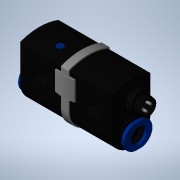
# Autodesk Inventor part: 527458 SDE5-Q6-M8(O)---(DS)
Saved by Autodesk Inventor 2021 (Build 250183000, 183)
## iProperties
Created: 2026-04-21
Part Number: 527458 SDE5-Q6-M8(O)---(DS)
Material: Generic
Catalog Web Link: www.3dfindit.com
Description: SDE5-(DS)-Pressure sensors - Housing
Vendor: FESTO
Document SubType Name: Modeling
Designer: psAdmin
Manufacturer: FESTO
Mass: 14.2277 g
Surface Area: 44.8821 cm^2
Volume: 14.2277 cm^3
Density: 1 g/cm^3
Appearance: PSOLRGB-79-79-79
Category: PARTsolutions
Company: FESTO
Title: 527458 SDE5-Q6-M8(O)---(DS)
Author: Cadenas PARTsolutions
Comments: Pressure sensors - Housing
PSOL_IDENT_0: {$CADENAS_DATA/23d-libs/festo/parts/s/sde5/parts/sde5.prj},216 {VTYP=3D},{NB=527458 SDE5-Q6-M8(O)---
PSOL_IDENT_1: (DS)},{LINA=527458 SDE5-Q6-M8(O)---(DS)},{NN=SDE5-(DS)},{DATE=22.08.2025 13:16:38},{GEOMDATE=30.08.2
PSOL_IDENT_2: 023 07:21:38},{VERSION=},{LINEID=110},{WBVAR=SF,PA,EAN,WSEX},{WBNUMERIC=WSEX}  {NB=527458 SDE5-Q6-M8
PSOL_IDENT_3: (O)---(DS)},{LINA=527458 SDE5-Q6-M8(O)---(DS)},{KT=DUMMY},{TNR=527458},{TYP=SDE5},{SF=O},{PA=Q6},{EA
PSOL_IDENT_4: N=M8},{PA1='Q6'},{PAN=1},{EA=P},{EAN1='M8'},{AK1=''},{VERS=11.000},{QST=3.1},{QSD=6},{EANX=2},{WSEX=
PSOL_IDENT_5: 0.000},{WSEX1=0.000},{WSEX2=}
NB: 527458 SDE5-Q6-M8(O)---(DS)
NN: SDE5-(DS)
NT: Pressure sensors - Housing
NBSYN: $TNR. $TYP.-$PA.-$EAN.($SF.)$WSEX2.---(DS)
LINA: 527458 SDE5-Q6-M8(O)---(DS)
CATALOG: Festo
TNR: 527458
TYP: SDE5
SF: O
PA: Q6
EAN: M8
EA: P
WSEX: 0
SUPPLIER: FESTO
ARTICLENO: 527458 SDE5-Q6-M8(O)---(DS)
BOMINFO: 527458 SDE5-Q6-M8(O)---(DS)
CREATOR: CADENAS GmbH
Autodesk Inventor part; units mm, degrees
sketch "Skizze_1" plane through (0, 0, 0) normal (1, 0, 0) x (0, 1, 0)
  arc A0 (8, 8) -> (8, -8) centre (8, 0) ccw
  line L0 (8, -8) -> (22.6494, -8)
  arc A1 (22.6494, -8) -> (23.118, -7.6744) centre (22.6494, -7.5) ccw
  arc A2 (23.118, -7.6744) -> (23.118, 7.6744) centre (2.5, 0) ccw
  arc A3 (23.118, 7.6744) -> (22.6494, 8) centre (22.6494, 7.5) ccw
  line L1 (22.6494, 8) -> (8, 8)
  constraints: 8 point on circle, 4 centre point, 4 end point
extrude "Extrusion1" add sketch "Skizze_1" along normal mid plane 38.5
sketch "Skizze_2" plane through (0, 0, 0) normal (0, 1, 0) x (-1, 0, 0)
  line L0 (0, -18) -> (0, -8)
  line L1 (0, -8) -> (-18.75, -8)
  arc A0 (-19.25, -7.5) -> (-18.75, -8) centre (-18.75, -7.5) ccw
  line L2 (-19.25, -7.5) -> (-19.25, 7.5)
  arc A1 (-18.75, 8) -> (-19.25, 7.5) centre (-18.75, 7.5) ccw
  line L3 (-18.75, 8) -> (0, 8)
  line L4 (0, 8) -> (0, 18)
  line L5 (0, 18) -> (-29.25, 18)
  line L6 (-29.25, 18) -> (-29.25, -18)
  line L7 (-29.25, -18) -> (0, -18)
  constraints: 16 end point, 4 point on circle, 2 centre point
extrude "Extrusion2" cut sketch "Skizze_2" along normal blind 25
sketch "Skizze_3" plane through (0, 0, 0) normal (0, 1, 0) x (-1, 0, 0)
  line L0 (29.25, -18) -> (29.25, 18)
  line L1 (29.25, 18) -> (0, 18)
  line L2 (0, 18) -> (0, 8)
  line L3 (0, 8) -> (18.75, 8)
  arc A0 (19.25, 7.5) -> (18.75, 8) centre (18.75, 7.5) ccw
  line L4 (19.25, 7.5) -> (19.25, -7.5)
  arc A1 (18.75, -8) -> (19.25, -7.5) centre (18.75, -7.5) ccw
  line L5 (18.75, -8) -> (0, -8)
  line L6 (0, -8) -> (0, -18)
  line L7 (0, -18) -> (29.25, -18)
  constraints: 16 end point, 4 point on circle, 2 centre point
extrude "Extrusion3" cut sketch "Skizze_3" along normal blind 25
sketch "Skizze_4" plane through (0, 0, 0) normal (0, 0, 1) x (1, 0, 0)
  line L0 (-2, 8) -> (2, 8)
  line L1 (-25, 3) -> (-25, -5.0034)
  line L2 (-25, -5.0034) -> (-14, -5.0034)
  line L3 (-14, -5.0034) -> (-14, 0)
  line L4 (-14, 0) -> (-18.75, 0)
  arc A0 (-19.25, 0.5) -> (-18.75, 0) centre (-18.75, 0.5) ccw
  line L5 (-19.25, 0.5) -> (-19.25, 3)
  line L6 (-19.25, 3) -> (-25, 3)
  constraints: 14 end point, 2 point on circle, 1 centre point
revolve "Revolution1" cut sketch "Skizze_4" angle 180 mid plane about axis through (-2, 8, 0) along (1, 0, 0)
sketch "Skizze_5" plane through (0, 0, 0) normal (0, 0, 1) x (1, 0, 0)
  line L0 (-2, 8) -> (2, 8)
  line L1 (14, -5.0034) -> (25, -5.0034)
  line L2 (25, -5.0034) -> (25, 3)
  line L3 (25, 3) -> (19.25, 3)
  line L4 (19.25, 3) -> (19.25, 0.5)
  arc A0 (18.75, 0) -> (19.25, 0.5) centre (18.75, 0.5) ccw
  line L5 (18.75, 0) -> (14, 0)
  line L6 (14, 0) -> (14, -5.0034)
  constraints: 14 end point, 2 point on circle, 1 centre point
revolve "Revolution2" cut sketch "Skizze_5" angle 180 mid plane about axis through (-2, 8, 0) along (1, 0, 0)
sketch "Skizze_6" plane through (0, 0, 0) normal (0, 0, 1) x (1, 0, 0)
  line L0 (-19.25, 2.5) -> (-24.25, 2.5)
  line L1 (-24.25, 29.5) -> (-24.25, 22.5)
  line L2 (-24.25, 22.5) -> (-19.25, 22.5)
  line L3 (-19.25, 22.5) -> (-19.25, 24)
  arc A0 (-18.75, 24.5) -> (-19.25, 24) centre (-18.75, 24) ccw
  line L4 (-18.75, 24.5) -> (-18.75, 29.5)
  line L5 (-18.75, 29.5) -> (-24.25, 29.5)
  constraints: 12 end point, 2 point on circle, 1 centre point
revolve "Revolution3" cut sketch "Skizze_6" angle 90 mid plane about axis through (-19.25, 2.5, 0) along (-1, 0, 0)
sketch "Skizze_7" plane through (0, 0, 0) normal (0, 0, 1) x (1, 0, 0)
  line L0 (24.25, 2.5) -> (19.25, 2.5)
  arc A0 (19.25, 24) -> (18.75, 24.5) centre (18.75, 24) ccw
  line L1 (19.25, 24) -> (19.25, 22.5)
  line L2 (19.25, 22.5) -> (24.25, 22.5)
  line L3 (24.25, 22.5) -> (24.25, 29.5)
  line L4 (24.25, 29.5) -> (18.75, 29.5)
  line L5 (18.75, 29.5) -> (18.75, 24.5)
  constraints: 12 end point, 2 point on circle, 1 centre point
revolve "Revolution4" cut sketch "Skizze_7" angle 90 mid plane about axis through (24.25, 2.5, 0) along (-1, 0, 0)
sketch "Skizze_8" plane through (-13.7, 0, 0) normal (1, 0, 0) x (0, 0, -1)
  line L0 (-10, 17) -> (-10, 10)
  line L1 (-10, 10) -> (-8, 10)
  line L2 (-8, 10) -> (-8, 12.0163)
  arc A0 (-7.6294, 12.4993) -> (-8, 12.0163) centre (-7.5, 12.0163) ccw
  line L3 (-7.6294, 12.4993) -> (-6.4224, 12.8227)
  arc A1 (-6.4224, 12.8227) -> (-6.2, 13.1125) centre (-6.5, 13.1125) ccw
  line L4 (-6.2, 13.1125) -> (-6.2, 14.8875)
  arc A2 (-6.2, 14.8875) -> (-6.4224, 15.1773) centre (-6.5, 14.8875) ccw
  line L5 (-6.4224, 15.1773) -> (-7.6294, 15.5007)
  arc A3 (-8, 15.9837) -> (-7.6294, 15.5007) centre (-7.5, 15.9837) ccw
  line L6 (-8, 15.9837) -> (-8, 17)
  line L7 (-8, 17) -> (-10, 17)
  constraints: 16 end point, 8 point on circle, 4 centre point
extrude "Extrusion4" cut sketch "Skizze_8" along normal blind 5.3
sketch "Skizze_9" plane through (-13.7, 0, 0) normal (1, 0, 0) x (0, 0, -1)
  line L0 (6.2, 14.8875) -> (6.2, 13.1125)
  arc A0 (6.2, 13.1125) -> (6.4224, 12.8227) centre (6.5, 13.1125) ccw
  line L1 (6.4224, 12.8227) -> (7.6294, 12.4993)
  arc A1 (8, 12.0163) -> (7.6294, 12.4993) centre (7.5, 12.0163) ccw
  line L2 (8, 12.0163) -> (8, 10)
  line L3 (8, 10) -> (10, 10)
  line L4 (10, 10) -> (10, 17)
  line L5 (10, 17) -> (8, 17)
  line L6 (8, 17) -> (8, 15.9837)
  arc A2 (7.6294, 15.5007) -> (8, 15.9837) centre (7.5, 15.9837) ccw
  line L7 (7.6294, 15.5007) -> (6.4224, 15.1773)
  arc A3 (6.4224, 15.1773) -> (6.2, 14.8875) centre (6.5, 14.8875) ccw
  constraints: 16 end point, 8 point on circle, 4 centre point
extrude "Extrusion5" cut sketch "Skizze_9" along normal blind 5.3
sketch "Skizze_10" plane through (13.7, 0, 0) normal (1, 0, 0) x (0, 0, -1)
  line L0 (-10, 17) -> (-10, 10)
  line L1 (-10, 10) -> (-8, 10)
  line L2 (-8, 10) -> (-8, 12.0163)
  arc A0 (-7.6294, 12.4993) -> (-8, 12.0163) centre (-7.5, 12.0163) ccw
  line L3 (-7.6294, 12.4993) -> (-6.4224, 12.8227)
  arc A1 (-6.4224, 12.8227) -> (-6.2, 13.1125) centre (-6.5, 13.1125) ccw
  line L4 (-6.2, 13.1125) -> (-6.2, 14.8875)
  arc A2 (-6.2, 14.8875) -> (-6.4224, 15.1773) centre (-6.5, 14.8875) ccw
  line L5 (-6.4224, 15.1773) -> (-7.6294, 15.5007)
  arc A3 (-8, 15.9837) -> (-7.6294, 15.5007) centre (-7.5, 15.9837) ccw
  line L6 (-8, 15.9837) -> (-8, 17)
  line L7 (-8, 17) -> (-10, 17)
  constraints: 16 end point, 8 point on circle, 4 centre point
extrude "Extrusion6" cut sketch "Skizze_10" against normal blind 5.3
sketch "Skizze_11" plane through (13.7, 0, 0) normal (1, 0, 0) x (0, 0, -1)
  line L0 (6.2, 14.8875) -> (6.2, 13.1125)
  arc A0 (6.2, 13.1125) -> (6.4224, 12.8227) centre (6.5, 13.1125) ccw
  line L1 (6.4224, 12.8227) -> (7.6294, 12.4993)
  arc A1 (8, 12.0163) -> (7.6294, 12.4993) centre (7.5, 12.0163) ccw
  line L2 (8, 12.0163) -> (8, 10)
  line L3 (8, 10) -> (10, 10)
  line L4 (10, 10) -> (10, 17)
  line L5 (10, 17) -> (8, 17)
  line L6 (8, 17) -> (8, 15.9837)
  arc A2 (7.6294, 15.5007) -> (8, 15.9837) centre (7.5, 15.9837) ccw
  line L7 (7.6294, 15.5007) -> (6.4224, 15.1773)
  arc A3 (6.4224, 15.1773) -> (6.2, 14.8875) centre (6.5, 14.8875) ccw
  constraints: 16 end point, 8 point on circle, 4 centre point
extrude "Extrusion7" cut sketch "Skizze_11" against normal blind 5.3
sketch "Skizze_12" plane through (0, 0, 0) normal (1, 0, 0) x (0, 1, 0)
  arc A0 (8, 8.5) -> (8, -8.5) centre (8, 0) ccw
  line L0 (8, -8.5) -> (22.9939, -8.5)
  arc A1 (22.9939, -8.5) -> (23.4597, -8.1818) centre (22.9939, -8) ccw
  arc A2 (23.4597, -8.1818) -> (23.4597, 8.1818) centre (2.5, 0) ccw
  arc A3 (23.4597, 8.1818) -> (22.9939, 8.5) centre (22.9939, 8) ccw
  line L1 (22.9939, 8.5) -> (8, 8.5)
  constraints: 8 point on circle, 4 centre point, 4 end point
extrude "Extrusion8" add sketch "Skizze_12" along normal mid plane 3.1
sketch "Sketch_14" plane through (0, 0, 0) normal (0, 0, 1) x (1, 0, 0)
  line L0 (22.35, 6) -> (19.25, 6)
  line L1 (19.25, 9.1) -> (21.35, 9.1)
  line L2 (21.35, 9.1) -> (22.1028, 9.2347)
  arc A0 (22.1028, 9.2347) -> (22.3454, 9.5821) centre (22.05, 9.53) ccw
  line L3 (22.3454, 9.5821) -> (21.9367, 11.9)
  line L4 (21.9367, 11.9) -> (20.85, 11.9)
  line L5 (20.85, 11.9) -> (20.85, 9.5)
  line L6 (20.85, 9.5) -> (20.05, 9.5)
  line L7 (20.05, 9.5) -> (20.05, 10.8)
  line L8 (20.05, 10.8) -> (19.85, 11)
  line L9 (19.85, 11) -> (19.25, 11)
  line L10 (19.25, 11) -> (19.25, 9.1)
  constraints: 22 end point, 2 point on circle, 1 centre point
revolve "Revolution5" add sketch "Sketch_14" angle 360 about axis through (22.35, 6, 0) along (1, 0, 0)
sketch "Sketch_15" plane through (22.45, 0, 0) normal (1, 0, 0) x (0, 0, -1)
  line L0 (-7, 0) -> (7, 0)
  line L1 (7, 0) -> (7, 12)
  line L2 (7, 12) -> (-7, 12)
  line L3 (-7, 12) -> (-7, 0)
  arc A0 (-1, 10.9) -> (-1, 1.1) centre (-1, 6) ccw
  line L4 (-1, 1.1) -> (1, 1.1)
  arc A1 (1, 1.1) -> (1, 10.9) centre (1, 6) ccw
  line L5 (1, 10.9) -> (-1, 10.9)
  constraints: 12 end point, 4 point on circle, 2 centre point
extrude "Extrusion9" cut sketch "Sketch_15" along normal mid plane 4
sketch "Sketch_16" plane through (0, 0, 0) normal (0, 0, 1) x (1, 0, 0)
  line L0 (-19.25, 6) -> (-22.35, 6)
  arc A0 (-22.3454, 9.5821) -> (-22.1028, 9.2347) centre (-22.05, 9.53) ccw
  line L1 (-22.1028, 9.2347) -> (-21.35, 9.1)
  line L2 (-21.35, 9.1) -> (-19.25, 9.1)
  line L3 (-19.25, 9.1) -> (-19.25, 11)
  line L4 (-19.25, 11) -> (-19.85, 11)
  line L5 (-19.85, 11) -> (-20.05, 10.8)
  line L6 (-20.05, 10.8) -> (-20.05, 9.5)
  line L7 (-20.05, 9.5) -> (-20.85, 9.5)
  line L8 (-20.85, 9.5) -> (-20.85, 11.9)
  line L9 (-20.85, 11.9) -> (-21.9367, 11.9)
  line L10 (-21.9367, 11.9) -> (-22.3454, 9.5821)
  constraints: 22 end point, 2 point on circle, 1 centre point
revolve "Revolution6" add sketch "Sketch_16" angle 360 about axis through (-19.25, 6, 0) along (1, 0, 0)
sketch "Sketch_17" plane through (-22.45, 0, 0) normal (1, 0, 0) x (0, 0, -1)
  line L0 (-7, 0) -> (7, 0)
  line L1 (7, 0) -> (7, 12)
  line L2 (7, 12) -> (-7, 12)
  line L3 (-7, 12) -> (-7, 0)
  arc A0 (-1, 10.9) -> (-1, 1.1) centre (-1, 6) ccw
  line L4 (-1, 1.1) -> (1, 1.1)
  arc A1 (1, 1.1) -> (1, 10.9) centre (1, 6) ccw
  line L5 (1, 10.9) -> (-1, 10.9)
  constraints: 12 end point, 4 point on circle, 2 centre point
extrude "Extrusion10" cut sketch "Sketch_17" along normal mid plane 4
sketch "Skizze_15" plane through (0, 17, 0) normal (0, 1, 0) x (1, 0, 0)
  line L0 (-4, -8) -> (-4, -8.5)
  arc A0 (-4, -8.5) -> (4, -8.5) centre (0, 7.25) ccw
  line L1 (4, -8.5) -> (4, -8)
  line L2 (4, -8) -> (-4, -8)
  constraints: 6 end point, 2 point on circle, 1 centre point
extrude "Extrusion11" add sketch "Skizze_15" along normal mid plane 8
sketch "Skizze_16" plane through (0, 17, 0) normal (0, 1, 0) x (1, 0, 0)
  line L0 (-4, 8) -> (4, 8)
  line L1 (4, 8) -> (4, 8.5)
  arc A0 (4, 8.5) -> (-4, 8.5) centre (0, -7.25) ccw
  line L2 (-4, 8.5) -> (-4, 8)
  constraints: 6 end point, 2 point on circle, 1 centre point
extrude "Extrusion12" add sketch "Skizze_16" along normal mid plane 8
sketch "Skizze_17" plane through (0, 0, 0) normal (0, 0, 1) x (1, 0, 0)
  line L0 (26.25, 18) -> (19.25, 18)
  line L1 (19.25, 18) -> (19.25, 20.9)
  line L2 (19.25, 20.9) -> (19.55, 20.9)
  line L3 (19.55, 20.9) -> (19.55, 21.25)
  line L4 (19.55, 21.25) -> (24.4264, 21.25)
  line L5 (24.4264, 21.25) -> (24.48, 21.45)
  line L6 (24.48, 21.45) -> (24.63, 21.45)
  line L7 (24.63, 21.45) -> (26.1031, 21.2482)
  arc A0 (26.25, 21.0798) -> (26.1031, 21.2482) centre (26.08, 21.0798) ccw
  line L8 (26.25, 21.0798) -> (26.0702, 20.9)
  line L9 (26.0702, 20.9) -> (21.25, 20.9)
  line L10 (21.25, 20.9) -> (21.25, 18)
  line L11 (21.25, 18) -> (19.25, 18)
  constraints: 24 end point, 2 point on circle, 1 centre point
revolve "Revolution7" add sketch "Skizze_17" angle 360 about axis through (26.25, 18, 0) along (1, 0, 0)
sketch "Sketch_2" plane through (0, 0, 0) normal (0, 0, 1) x (1, 0, 0)
  line L0 (23.25, 18) -> (20.25, 18)
  line L1 (20.25, 21) -> (23.25, 21)
  line L2 (23.25, 21) -> (23.25, 21.7)
  line L3 (23.25, 21.7) -> (22.95, 22)
  line L4 (22.95, 22) -> (20.75, 22)
  line L5 (20.75, 22) -> (20.25, 21.5)
  line L6 (20.25, 21.5) -> (20.25, 21)
  constraints: 14 end point
revolve "Revolution8" add sketch "Sketch_2" angle 360 about axis through (23.25, 18, 0) along (1, 0, 0)
thread "Thread1" size "M8x1" class "6g" standard "ISO Metric profile" full length
sketch "Sketch_3" plane through (0, 18, 0) normal (0, 1, 0) x (1, 0, 0)
  line L0 (25.75, 1.75) -> (21.25, 1.75)
  line L1 (21.25, 1.75) -> (21.25, 2.25)
  line L2 (21.25, 2.25) -> (25.25, 2.25)
  arc A0 (25.75, 1.75) -> (25.25, 2.25) centre (25.25, 1.75) ccw
  line L3 (25.75, 1.75) -> (21.25, 1.75)
  constraints: 8 end point, 2 point on circle, 1 centre point
revolve "Revolution9" add sketch "Sketch_3" angle 360 about axis through (25.75, 18, -1.75) along (1, 0, 0)
sketch "Sketch_4" plane through (0, 18, 0) normal (0, 1, 0) x (1, 0, 0)
  line L0 (25.75, -1.75) -> (21.25, -1.75)
  line L1 (21.25, -1.75) -> (21.25, -1.25)
  line L2 (21.25, -1.25) -> (25.25, -1.25)
  arc A0 (25.75, -1.75) -> (25.25, -1.25) centre (25.25, -1.75) ccw
  line L3 (25.75, -1.75) -> (21.25, -1.75)
  constraints: 8 end point, 2 point on circle, 1 centre point
revolve "Revolution10" add sketch "Sketch_4" angle 360 about axis through (25.75, 18, 1.75) along (1, 0, 0)
sketch "Sketch_7" plane through (0, 18, 0) normal (0, 0, 1) x (1, 0, 0)
  line L0 (25.75, -1.75) -> (21.25, -1.75)
  line L1 (21.25, -1.75) -> (21.25, -1.25)
  line L2 (21.25, -1.25) -> (25.25, -1.25)
  arc A0 (25.75, -1.75) -> (25.25, -1.25) centre (25.25, -1.75) ccw
  line L3 (25.75, -1.75) -> (21.25, -1.75)
  constraints: 8 end point, 2 point on circle, 1 centre point
revolve "Revolution11" add sketch "Sketch_7" angle 360 about axis through (25.75, 16.25, 0) along (1, 0, 0)
sketch "Sketch_24" plane through (0, 0, 2.3) normal (0, 0, 1) x (1, 0, 0)
  line L0 (-8, 22) -> (-8, 27)
  line L1 (-8, 27) -> (-6.55, 27)
  line L2 (-6.55, 27) -> (-6.55, 22)
  line L3 (-6.55, 22) -> (-8, 22)
  line L4 (-8, 22) -> (-8, 27)
  constraints: 10 end point
revolve "Revolution12" cut sketch "Sketch_24" angle 360 about axis through (-8, 22, 2.3) along (0, -1, 0)
sketch "Sketch_25" plane through (0, 0, 2.3) normal (0, 0, 1) x (1, 0, 0)
  line L0 (-8, 22) -> (-8, 24.3)
  arc A0 (-8, 24.3) -> (-7, 24.4) centre (-8.2945, 32.2946) ccw
  line L1 (-7, 24.4) -> (-6.8, 24.4)
  arc A1 (-6.6, 24.2) -> (-6.8, 24.4) centre (-6.8, 24.2) ccw
  line L2 (-6.6, 24.2) -> (-6.6, 22)
  line L3 (-6.6, 22) -> (-8, 22)
  line L4 (-8, 22) -> (-8, 24.3)
  constraints: 10 end point, 4 point on circle, 2 centre point
revolve "Revolution13" add sketch "Sketch_25" angle 360 about axis through (-8, 22, 2.3) along (0, -1, 0)
ref_plane "CLIP_XY" through (0, 8, 0) normal (1, 0, 0) x (0, 0, -1)
ref_plane "CLIP_YZ" through (0, 8, 0) normal (0, 0, -1) x (0, 1, 0)
ref_plane "CLIP_ZX" through (0, 8, 0) normal (0, 1, 0) x (1, 0, 0)
ref_plane "TO_DUMMY_XY" through (0, 0, 0) normal (0, -1, 0) x (0, 0, 1)
ref_plane "TO_DUMMY_YZ" through (0, 0, 0) normal (0, 0, 1) x (-1, 0, 0)
ref_plane "TO_DUMMY_ZX" through (0, 0, 0) normal (-1, 0, 0) x (0, -1, 0)
ref_plane "TO_NEBU_XY" through (20.1, 18, 0) normal (1, 0, 0) x (0, 0, -1)
ref_plane "TO_NEBU_YZ" through (20.1, 18, 0) normal (0, 0, -1) x (0, 1, 0)
ref_plane "TO_NEBU_ZX" through (20.1, 18, 0) normal (0, 1, 0) x (1, 0, 0)
body "Solid1"
